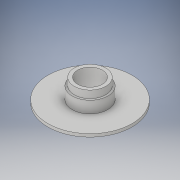
# Autodesk Inventor part: Part4
Saved by Autodesk Inventor 2019 (Build 230136000, 136)
## iProperties
Created: 2020-02-28
Part Number: Part4
Material: Generic
Document SubType Name: Modeling
Designer: gfb14170
Density: 1 g/cm^3
Appearance: Default
Author: gfb14170
Autodesk Inventor part; units mm, degrees
ref_plane "YZ Plane" through (0, 0, 0) normal (1, 0, 0) x (0, 1, 0)
ref_plane "XZ Plane" through (0, 0, 0) normal (0, 1, 0) x (-1, 0, 0)
ref_plane "XY Plane" through (0, 0, 0) normal (0, 0, 1) x (1, 0, 0)
sketch "Sketch1" plane through (0, 0, 0) normal (1, 0, 0) x (0, 1, 0)
  line L0 (11.25, 0) -> (-11.25, 0) construction
  line L1 (-11.25, 12.5) -> (11.25, 12.5)
  line L2 (11.25, 0) -> (-11.25, 0)
  line L3 (-11.25, 12.5) -> (-11.25, 16)
  line L4 (-11.25, 16) -> (11.25, 16)
  line L5 (11.25, 16) -> (11.25, 12.5)
  line L6 (-11.25, 16) -> (3.75, 16)
  line L7 (3.75, 16) -> (3.75, 18)
  line L8 (3.75, 18) -> (-11.25, 18)
  line L9 (-11.25, 18) -> (-11.25, 16)
  line L10 (-11.25, 18) -> (-8.25, 18)
  line L11 (-8.25, 18) -> (-8.25, 42.5)
  line L12 (-8.25, 42.5) -> (-11.25, 42.5)
  line L13 (-11.25, 42.5) -> (-11.25, 18)
  point P0 (0, 0)
  dimension "d0" = 12.5
  dimension "d1" = 0
  dimension "d2" = 22.5
  dimension "d3" = 16
  dimension "d6" = 18
  dimension "d7" = 7.5
  dimension "d8" = 42.5
  dimension "d10" = 11.25
  dimension "d11" = 19.5
  constraints: 28 end point, 7 parallel, 4 horizontal, 3 perpendicular
  measures "d0" distance between parallel lines of L0 L1
  measures "d1" distance from line of point (0, 0) L0
  measures "d2" distance of L3.end L4.end
  measures "d3" distance between parallel lines of L0 L4
  measures "d6" distance from line of L8 point (0, 0)
  measures "d7" distance between parallel lines of L7 L5
  measures "d8" distance from line of point (0, 0) L12
  measures "d10" distance from line of point (0, 0) L5
  measures "d11" distance between parallel lines of L11 L5
revolve "Revolution1" add sketch "Sketch1" angle 360 about axis through (0, 11.25, 0) along (0, -1, 0)
equation "\"d2\" = d4 + d5"
equation "\"d5\" = d4"
equation "\"d4\" = 11.25"
body "Solid1"
